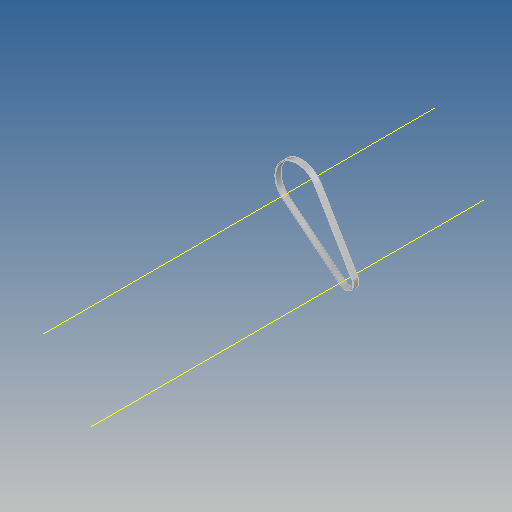
# Autodesk Inventor part: Synchronous Belt
Saved by Autodesk Inventor 2020 (Build 240168000, 168)
## iProperties
CustomPartVersion: 1
Created: 2021-06-15
Part Number: Synchronous Belt
Material: Rubber
Document SubType Name: Modeling
Designer: Iulian Bors
Density: 0.93 g/cm^3
Appearance: Rubber - Black - Version 1.1
Mass: 0.402996 g
Surface Area: 16.611 cm^2
Volume: 0.43333 cm^3
Author: Iulian Bors
Subject: 1100
Autodesk Inventor part; units mm, degrees
sketch "Sketch Path" plane through (0, 0, 0) normal (0, 0, 1) x (1, 0, 0)
  arc A0 (-8.3588, 1.2274) -> (0.4994, 8.9316) centre (-4.638, 5.8939) ccw
  arc A1 (-27.0318, 55.4943) -> (-50.6536, 34.9498) centre (-40.7317, 47.3939) ccw
  line L0 (-27.0318, 55.4943) -> (0.4994, 8.9316)
  line L1 (-8.3588, 1.2274) -> (-50.6536, 34.9498)
  constraints: 4 end point, 4 point on circle, 2 centre point
ref_plane "Cross Section Plane" through (0.4994, 8.9316, 0) normal (-0.509, 0.8608, 0) x (0, 0, 1)
ref_plane "Work Plane2" through (-4.638, 5.8939, 0) normal (-1, 0, 0) x (0, 0, 1)
ref_plane "Work Plane3" through (-40.7317, 47.3939, 0) normal (0.7562, -0.6543, 0) x (0, 0, 1)
sketch "Cross Section" plane through (0.4994, 8.9316, 0) normal (-0.509, 0.8608, 0) x (0, 0, 1)
  line L0 (-2, 0.3) -> (2, 0.3)
  line L1 (2, 0.3) -> (2, -0.3)
  line L2 (2, -0.3) -> (-2, -0.3)
  line L3 (-2, -0.3) -> (-2, 0.3)
  line L4 (-2, 0) -> (2, 0) construction
  point P0 (0, 0)
  point P1 (0, 0)
  dimension "d0" = 4
  dimension "d4" = 0.3
  dimension "d5" = 0.3
  constraints: 10 end point, 3 midpoint, 2 parallel, 1 coincident, 1 horizontal, 1 perpendicular, 1 other
  measures "d0" distance between parallel lines of L1 L3
  measures "d4" distance between parallel lines of L2 L4
  measures "d5" distance between parallel lines of L4 L0
sweep "Belt" add profiles "Cross Section" path "Sketch Path"
equation "\"d0\" = da_B"
equation "\"d4\" = da_a"
equation "\"d5\" = da_a2"
equation "\"da_B\" = 4"
equation "\"da_pb\" = 2.5"
equation "\"da_L\" = 180.55398"
equation "\"da_a\" = 0.3"
equation "\"da_S\" = 1.5"
equation "\"da_Beta\" = 20deg"
equation "\"da_Ht\" = 0.7"
equation "\"da_H\" = 1.3"
equation "\"da_a2\" = 0.3"
body "Solid1"
